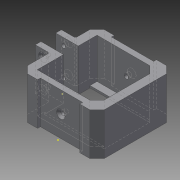
# Autodesk Inventor part: Stepper mount v1
Saved by Autodesk Inventor 2015 (Build 190159000, 159)
## iProperties
Created: 2019-01-11
Part Number: Stepper mount v1
Material: Generic
Document SubType Name: Modeling
Designer: Toby
Density: 1 g/cm^3
Appearance: Default
Author: Toby
Autodesk Inventor part; units mm, degrees
ref_plane "YZ Plane" through (0, 0, 0) normal (1, 0, 0) x (0, 1, 0)
ref_plane "XZ Plane" through (0, 0, 0) normal (0, 1, 0) x (-1, 0, 0)
ref_plane "XY Plane" through (0, 0, 0) normal (0, 0, 1) x (1, 0, 0)
sketch "Sketch1" plane through (0, 0, 0) normal (0, 0, 1) x (1, 0, 0)
  line L0 (-20.7464, 18.5829) -> (21.7536, 18.5829)
  line L1 (21.7536, 18.5829) -> (21.7536, -23.9171)
  line L2 (21.7536, -23.9171) -> (-20.7464, -23.9171)
  line L3 (-20.7464, -23.9171) -> (-20.7464, 18.5829)
  line L4 (-26.7464, 24.5829) -> (27.7536, 24.5829)
  line L5 (27.7536, 24.5829) -> (27.7536, -29.9171)
  line L6 (27.7536, -29.9171) -> (-26.7464, -29.9171)
  line L7 (-26.7464, -29.9171) -> (-26.7464, 24.5829)
  point P0 (0, 0)
  dimension "d0" = 42.5
  dimension "d1" = 42.5
  dimension "d2" = 6
  dimension "d3" = 6
  dimension "d4" = 6
  dimension "d5" = 6
  constraints: 16 end point, 4 parallel, 2 horizontal, 2 perpendicular
  measures "d0" distance of L0.end L1.end
  measures "d1" distance of L0.start L0.end
  measures "d2" distance between parallel lines of L0 L4
  measures "d3" distance between parallel lines of L6 L2
  measures "d4" distance between parallel lines of L5 L1
  measures "d5" distance between parallel lines of L3 L7
extrude "Extrusion1" add sketch "Sketch1" along normal blind 30
chamfer "Chamfer1" distance 5 angle 45 4 edges at (27.7536, 24.5829, 15) (27.7536, -29.9171, 15) (21.7536, -23.9171, 15) (21.7536, 18.5829, 15)
chamfer "Chamfer2" distance 5 angle 45 2 edges at (-26.7464, 24.5829, 15) (-26.7464, -29.9171, 15)
sketch "Sketch2" plane through (22.7536, -29.9171, 0) normal (0, -1, 0) x (1, 0, 0)
  line L0 (-44.5, 30) -> (0, 30) projected
  point P0 (-22.7536, 0)
  point P1 (-22.7536, 15)
  dimension "d14" = 15
  measures "d14" distance from line of L0 point (-22.754, 15)
hole "Hole1" at (0, -29.9171, 15) direction (0, 1, 0) diameter 3 depth 100 tip angle 118
sketch "Sketch3" plane through (0, 0, 30) normal (0, 0, 1) x (1, 0, 0)
  line L0 (-21.7464, -29.9171) -> (22.7536, -29.9171) projected
  line L1 (-14.4964, -29.9171) -> (15.5036, -29.9171)
  line L2 (15.5036, -29.9171) -> (15.5036, -27.9171)
  line L3 (15.5036, -27.9171) -> (-14.4964, -27.9171)
  line L4 (-14.4964, -27.9171) -> (-14.4964, -29.9171)
  line L5 (-21.7464, 24.5829) -> (22.7536, 24.5829) projected
  line L6 (-14.4964, 24.5829) -> (15.5036, 24.5829)
  line L7 (15.5036, 24.5829) -> (15.5036, 22.5829)
  line L8 (15.5036, 22.5829) -> (-14.4964, 22.5829)
  line L9 (-14.4964, 22.5829) -> (-14.4964, 24.5829)
  line L10 (-20.7464, -23.9171) -> (-20.7464, 18.5829) projected
  point P0 (0, 0)
  dimension "d22" = 30
  dimension "d23" = 6.25
  dimension "d24" = 2
  dimension "d25" = 2
  constraints: 16 end point, 4 parallel, 4 point on line, 2 horizontal, 2 perpendicular
  measures "d22" distance between parallel lines of L2 L4
  measures "d23" distance between parallel lines of L10 L4
  measures "d24" distance between parallel lines of L0 L3
  measures "d25" distance between parallel lines of L5 L8
extrude "Extrusion2" cut sketch "Sketch3" against normal blind 30
sketch "Sketch4" plane through (-26.7464, -24.9171, 0) normal (-1, 0, 0) x (0, 0, 1)
  point P0 (0, 24.9171)
sketch "Sketch5" plane through (-26.7464, -24.9171, 0) normal (-1, 0, 0) x (0, 0, 1)
  line L0 (30, 38.5) -> (30, 6) projected
  line L1 (30, 34.1671) -> (0, 34.1671)
  line L2 (0, 34.1671) -> (0, 30.1671)
  line L3 (0, 30.1671) -> (30, 30.1671)
  line L4 (30, 30.1671) -> (30, 34.1671)
  line L5 (30, 19.6671) -> (0, 19.6671)
  line L6 (0, 19.6671) -> (0, 15.6671)
  line L7 (0, 15.6671) -> (30, 15.6671)
  line L8 (30, 15.6671) -> (30, 19.6671)
  line L9 (0, 0) -> (0, 44.5) projected
  point P0 (0, 24.9171)
  dimension "d28" = 10.5
  dimension "d29" = 4
  dimension "d30" = 4
  dimension "d31" = 5.25
  constraints: 16 end point, 4 parallel, 3 point on line, 2 horizontal, 2 perpendicular, 1 collinear
  measures "d28" distance between parallel lines of L5 L3
  measures "d29" distance between parallel lines of L3 L1
  measures "d30" distance of L5.end L6.end
  measures "d31" distance from line of point (0, 24.917) L5
extrude "Extrusion3" add sketch "Sketch5" along normal blind 10 contours L0 L3 L2 L1 | L0 L7 L6 L5
sketch "Sketch6" plane through (22.7536, -29.9171, 0) normal (0, -1, 0) x (1, 0, 0)
  point P0 (-22.7536, 0)
sketch "Sketch7" plane through (-14.4964, -27.9171, 30) normal (0, -1, 0) x (1, 0, 0)
  circle A0 centre (14.4964, -15) radius 1.5 projected
  point P0 (14.4964, -30)
  constraints: 1 coincident
hole "Hole2" at (0, -27.9171, 15) direction (0, 1, 0) diameter 3 depth 100 tip angle 118 countersink diameter 6 countersink angle 90
sketch "Sketch8" plane through (-14.4964, 22.5829, 30) normal (0, 1, 0) x (1, 0, 0)
  circle A0 centre (14.4964, 15) radius 1.5 projected
  point P0 (14.4964, 30)
  constraints: 1 coincident
hole "Hole3" at (0, 22.5829, 15) direction (0, -1, 0) diameter 3 depth 5 tip angle 118 countersink diameter 6 countersink angle 90
sketch "Sketch9" plane through (-26.7464, -9.25, 0) normal (0, -1, 0) x (1, 0, 0)
  line L0 (0, 30) -> (-10, 30) projected
  line L1 (0, 0) -> (-10, 0) projected
  point P0 (26.7464, 0)
  point P1 (-4.7181, 25)
  point P2 (-4.7181, 5)
  dimension "d48" = 5
  dimension "d49" = 5
  measures "d48" distance from line of L0 point (-4.718, 25)
  measures "d49" distance from line of L1 point (-4.718, 5)
hole "Hole4" at (-31.4645, -9.25, 25) at (-31.4645, -9.25, 5) direction (0, 1, 0) diameter 3 depth 5 tip angle 118 countersink diameter 6 countersink angle 90
sketch "Sketch10" plane through (-26.7464, 9.25, 30) normal (0, 1, 0) x (1, 0, 0)
  circle A0 centre (-4.7181, 5) radius 1.5 projected
  circle A1 centre (-4.7181, 25) radius 1.5 projected
  point P0 (26.7464, 30)
  constraints: 2 coincident
hole "Hole5" at (-31.4645, 9.25, 25) at (-31.4645, 9.25, 5) direction (0, -1, 0) diameter 3 depth 5 tip angle 118 countersink diameter 6 countersink angle 90
sketch "Sketch11" plane through (0, 0, 0) normal (0, 0, -1) x (-1, 0, 0)
  line L0 (-21.7536, 13.5829) -> (20.7464, 13.5829)
  line L1 (20.7464, 13.5829) -> (20.7464, 18.5829)
  line L2 (20.7464, 18.5829) -> (-21.7536, 18.5829)
  line L3 (-21.7536, 18.5829) -> (-21.7536, 13.5829)
  line L4 (20.7464, -23.9171) -> (-21.7536, -23.9171)
  line L5 (-21.7536, -23.9171) -> (-21.7536, -18.9171)
  line L6 (-21.7536, -18.9171) -> (20.7464, -18.9171)
  line L7 (20.7464, -18.9171) -> (20.7464, -23.9171)
  line L8 (20.7464, -23.9171) -> (-16.7536, -23.9171) projected
  point P0 (0, 0)
  dimension "d64" = 5
  constraints: 16 end point, 4 parallel, 2 horizontal, 2 perpendicular, 2 point on line, 1 collinear
  measures "d64" distance between parallel lines of L4 L6
extrude "Extrusion4" add sketch "Sketch11" against normal blind 1.5
sketch "Sketch12" plane through (-26.7464, -5.25, 0) normal (-1, 0, 0) x (0, 0, 1)
  point P0 (0, 5.25)
sketch "Sketch13" plane through (-26.7464, -5.25, 0) normal (-1, 0, 0) x (0, 0, 1)
  line L0 (30, 10.5) -> (0, 10.5)
  line L1 (0, 10.5) -> (0, 0)
  line L2 (0, 0) -> (30, 0)
  line L3 (30, 0) -> (30, 10.5)
  point P0 (0, 5.25)
  constraints: 8 end point, 2 parallel, 1 horizontal, 1 perpendicular
extrude "Extrusion5" cut sketch "Sketch13" against normal blind 6
chamfer "Chamfer3" distance 1 angle 45 1 edges at (-26.7464, 9.25, 15)
chamfer "Chamfer4" distance 1 angle 45 1 edges at (-26.7464, -9.25, 15)
body "Solid1"
